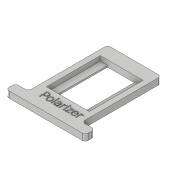
# Autodesk Inventor part: 00_Polarizationfilter_Holder
Saved by Autodesk Inventor 2019.4 (Build 234330000, 330)
## iProperties
Created: 2021-10-22
Part Number: 00_Polarizationfilter_Holder
Material: Generic
Document SubType Name: Modeling
Designer: diederichbenedict
Density: 1 g/cm^3
Appearance: Default
Author: diederichbenedict
Autodesk Inventor part; units mm, degrees
ref_plane "YZ Plane" through (0, 0, 0) normal (1, 0, 0) x (0, 1, 0)
ref_plane "XZ Plane" through (0, 0, 0) normal (0, 1, 0) x (-1, 0, 0)
ref_plane "XY Plane" through (0, 0, 0) normal (0, 0, 1) x (1, 0, 0)
sketch "Sketch1" plane through (0, 0, 0) normal (0, 1, 0) x (-1, 0, 0)
  line L0 (-16.92, 25) -> (16.92, 25)
  line L1 (16.92, 25) -> (16.92, -25)
  line L2 (16.92, -25) -> (-16.92, -25)
  line L3 (-16.92, -25) -> (-16.92, 25)
  line L4 (-16.92, 25) -> (16.92, -25) construction
  line L5 (16.92, 25) -> (-16.92, -25) construction
  line L6 (8.92, -17) -> (8.92, 17)
  line L7 (8.92, 17) -> (-8.92, 17)
  line L8 (-8.92, 17) -> (-8.92, -17)
  line L9 (-8.92, -17) -> (8.92, -17)
  line L10 (-25, 31) -> (25, 31)
  line L11 (25, 31) -> (25, 25)
  line L12 (25, 25) -> (-25, 25)
  line L13 (-25, 25) -> (-25, 31)
  line L14 (-25, 31) -> (25, 25) construction
  line L15 (25, 31) -> (-25, 25) construction
  point P0 (0, 0)
  point P1 (0, 28)
  point P2 (0, 25)
  dimension "d0" = 33.84
  dimension "d1" = 50
  dimension "d2" = 8
  dimension "d3" = 50
  dimension "d4" = 6
  constraints: 32 end point, 6 midpoint, 6 parallel, 3 perpendicular, 2 horizontal, 3 other
  measures "d0" distance of L1.end L2.end
  measures "d1" distance of L0.end L1.end
  measures "d2" distance between parallel lines of L1 L6
  measures "d3" distance of L11.end L12.end
  measures "d4" distance of L10.end L11.end
extrude "Extrusion1" add sketch "Sketch1" along normal blind 4
sketch "Sketch2" plane through (0, 4, 0) normal (0, 1, 0) x (1, 0, 0)
  line L0 (-8.92, 17) -> (8.92, 17) projected
  line L1 (8.92, 17) -> (8.92, -17) projected
  line L2 (8.92, -17) -> (-8.92, -17) projected
  line L3 (-8.92, -17) -> (-8.92, 17) projected
  line L4 (25, -25) -> (16.92, -25) projected
  line L5 (16.92, -25) -> (16.92, 25) projected
  line L6 (16.92, 25) -> (-16.92, 25) projected
  line L7 (-16.92, 25) -> (-16.92, -25) projected
  line L8 (-16.92, -25) -> (-25, -25) projected
  line L9 (-25, -25) -> (-25, -31) projected
  line L10 (-25, -31) -> (25, -31) projected
  line L11 (25, -31) -> (25, -25) projected
  line L12 (13.5, 17) -> (-13.5, 17)
  line L13 (-13.5, 17) -> (-13.5, -17)
  line L14 (-13.5, -17) -> (13.5, -17)
  line L15 (13.5, -17) -> (13.5, 17)
  line L16 (13.5, 17) -> (-13.5, -17) construction
  line L17 (-13.5, 17) -> (13.5, -17) construction
  point P0 (0, 0)
  dimension "d7" = 27
  dimension "d8" = 34
  constraints: 12 end point, 2 midpoint, 2 parallel, 1 horizontal, 1 perpendicular
  measures "d7" distance of L14.end L13.end
  measures "d8" distance of L13.end L12.end
extrude "Extrusion2" cut sketch "Sketch2" against normal blind 3 contours L3 L14 L13 L12 | L12 L15 L14 L1
sketch "Sketch3" plane through (0, 4, 0) normal (0, 1, 0) x (1, 0, 0)
  line L0 (-11.1728, -19.2539) -> (14.053, -19.2539) construction
  line L1 (14.053, -19.2539) -> (14.053, -24.441) construction
  line L2 (14.053, -24.441) -> (-11.1728, -24.441) construction
  line L3 (-11.1728, -24.441) -> (-11.1728, -19.2539) construction
  spline S0 degree 2 poles (-7.603, -20.9382) (-7.603, -21.2538) (-7.8278, -21.8218) (-8.029, -22.019) knots 0 0 0 1 2 2 2
  spline S1 degree 2 poles (-8.029, -22.019) (-8.2814, -22.2675) (-8.9639, -22.5239) (-9.4846, -22.5239) knots 0 0 0 1 2 2 2
  line L4 (-9.4846, -22.5239) -> (-10.0329, -22.5239)
  line L5 (-10.0329, -22.5239) -> (-10.0329, -24.3385)
  line L6 (-10.0329, -24.3385) -> (-10.6798, -24.3385)
  line L7 (-10.6798, -24.3385) -> (-10.6798, -19.4708)
  line L8 (-10.6798, -19.4708) -> (-9.4569, -19.4708)
  spline S2 degree 2 poles (-9.4569, -19.4708) (-9.023, -19.4708) (-8.4156, -19.6128) (-8.1828, -19.7745) knots 0 0 0 1 2 2 2
  spline S3 degree 2 poles (-8.1828, -19.7745) (-7.9107, -19.9599) (-7.603, -20.5319) (-7.603, -20.9382) knots 0 0 0 1 2 2 2
  spline S4 degree 2 poles (-8.2775, -20.9579) (-8.2775, -20.7055) (-8.4511, -20.3347) (-8.6286, -20.2163) knots 0 0 0 1 2 2 2
  spline S5 degree 2 poles (-8.6286, -20.2163) (-8.7824, -20.1138) (-9.1927, -20.0309) (-9.4964, -20.0309) knots 0 0 0 1 2 2 2
  line L9 (-9.4964, -20.0309) -> (-10.0329, -20.0309)
  line L10 (-10.0329, -20.0309) -> (-10.0329, -21.9717)
  line L11 (-10.0329, -21.9717) -> (-9.5911, -21.9717)
  spline S6 degree 2 poles (-9.5911, -21.9717) (-9.1966, -21.9717) (-8.7114, -21.8455) (-8.5536, -21.6798) knots 0 0 0 1 2 2 2
  spline S7 degree 2 poles (-8.5536, -21.6798) (-8.4077, -21.5338) (-8.2775, -21.1907) (-8.2775, -20.9579) knots 0 0 0 1 2 2 2
  spline S8 degree 2 poles (-4.0331, -22.5121) (-4.0331, -23.4351) (-4.9206, -24.441) (-5.6622, -24.441) knots 0 0 0 1 2 2 2
  spline S9 degree 2 poles (-5.6622, -24.441) (-6.4235, -24.441) (-7.2953, -23.4036) (-7.2953, -22.5121) knots 0 0 0 1 2 2 2
  spline S10 degree 2 poles (-7.2953, -22.5121) (-7.2953, -21.597) (-6.3959, -20.5832) (-5.6622, -20.5832) knots 0 0 0 1 2 2 2
  spline S11 degree 2 poles (-5.6622, -20.5832) (-4.9206, -20.5832) (-4.0331, -21.593) (-4.0331, -22.5121) knots 0 0 0 1 2 2 2
  spline S12 degree 2 poles (-4.6682, -22.5121) (-4.6682, -21.8021) (-5.1849, -21.1118) (-5.6622, -21.1118) knots 0 0 0 1 2 2 2
  spline S13 degree 2 poles (-5.6622, -21.1118) (-6.1395, -21.1118) (-6.6602, -21.8021) (-6.6602, -22.5121) knots 0 0 0 1 2 2 2
  spline S14 degree 2 poles (-6.6602, -22.5121) (-6.6602, -23.2024) (-6.1395, -23.9124) (-5.6622, -23.9124) knots 0 0 0 1 2 2 2
  spline S15 degree 2 poles (-5.6622, -23.9124) (-5.1889, -23.9124) (-4.6682, -23.2143) (-4.6682, -22.5121) knots 0 0 0 1 2 2 2
  line L12 (-2.7748, -24.3385) -> (-3.3901, -24.3385)
  line L13 (-3.3901, -24.3385) -> (-3.3901, -19.2539)
  line L14 (-3.3901, -19.2539) -> (-2.7748, -19.2539)
  line L15 (-2.7748, -19.2539) -> (-2.7748, -24.3385)
  spline S16 degree 2 poles (0.164, -23.9519) (0.089, -24.0071) (-0.1634, -24.2043) (-0.2818, -24.2635) knots 0 0 0 1 2 2 2
  spline S17 degree 2 poles (-0.2818, -24.2635) (-0.4435, -24.3503) (-0.7472, -24.441) (-1.0234, -24.441) knots 0 0 0 1 2 2 2
  spline S18 degree 2 poles (-1.0234, -24.441) (-1.2482, -24.441) (-1.6545, -24.2714) (-1.8083, -24.1176) knots 0 0 0 1 2 2 2
  spline S19 degree 2 poles (-1.8083, -24.1176) (-1.9543, -23.9677) (-2.1318, -23.5259) (-2.1318, -23.2813) knots 0 0 0 1 2 2 2
  spline S20 degree 2 poles (-2.1318, -23.2813) (-2.1318, -22.9026) (-1.8123, -22.3662) (-1.4651, -22.2123) knots 0 0 0 1 2 2 2
  spline S21 degree 2 poles (-1.4651, -22.2123) (-1.1575, -22.0703) (-0.3212, -21.9638) (0.164, -21.9362) knots 0 0 0 1 2 2 2
  line L16 (0.164, -21.9362) -> (0.164, -21.8179)
  spline S22 degree 2 poles (0.164, -21.8179) (0.164, -21.6048) (0.0338, -21.3406) (-0.0845, -21.2656) knots 0 0 0 1 2 2 2
  spline S23 degree 2 poles (-0.0845, -21.2656) (-0.2029, -21.1907) (-0.5421, -21.1433) (-0.7236, -21.1433) knots 0 0 0 1 2 2 2
  spline S24 degree 2 poles (-0.7236, -21.1433) (-0.9366, -21.1433) (-1.5125, -21.2696) (-1.8004, -21.3918) knots 0 0 0 1 2 2 2
  line L17 (-1.8004, -21.3918) -> (-1.8359, -21.3918)
  line L18 (-1.8359, -21.3918) -> (-1.8359, -20.7646)
  spline S25 degree 2 poles (-1.8359, -20.7646) (-1.6663, -20.7173) (-1.0312, -20.599) (-0.7196, -20.599) knots 0 0 0 1 2 2 2
  spline S26 degree 2 poles (-0.7196, -20.599) (-0.3409, -20.599) (0.1758, -20.7173) (0.3809, -20.8711) knots 0 0 0 1 2 2 2
  spline S27 degree 2 poles (0.3809, -20.8711) (0.5821, -21.021) (0.7793, -21.4983) (0.7793, -21.8415) knots 0 0 0 1 2 2 2
  line L19 (0.7793, -21.8415) -> (0.7793, -24.3385)
  line L20 (0.7793, -24.3385) -> (0.164, -24.3385)
  line L21 (0.164, -24.3385) -> (0.164, -23.9519)
  line L22 (0.164, -23.4391) -> (0.164, -22.4253)
  spline S28 degree 2 poles (0.164, -22.4253) (-0.0569, -22.4451) (-0.7236, -22.5121) (-0.9326, -22.5752) knots 0 0 0 1 2 2 2
  spline S29 degree 2 poles (-0.9326, -22.5752) (-1.1772, -22.6502) (-1.4967, -22.9618) (-1.4967, -23.2379) knots 0 0 0 1 2 2 2
  spline S30 degree 2 poles (-1.4967, -23.2379) (-1.4967, -23.5535) (-1.1417, -23.873) (-0.8025, -23.873) knots 0 0 0 1 2 2 2
  spline S31 degree 2 poles (-0.8025, -23.873) (-0.5145, -23.873) (-0.0411, -23.6245) (0.164, -23.4391) knots 0 0 0 1 2 2 2
  line L23 (3.58, -21.3445) -> (3.5485, -21.3445)
  spline S32 degree 2 poles (3.5485, -21.3445) (3.4775, -21.3248) (3.3236, -21.3169) (3.2171, -21.3169) knots 0 0 0 1 2 2 2
  spline S33 degree 2 poles (3.2171, -21.3169) (2.9686, -21.3169) (2.4795, -21.5338) (2.2586, -21.7469) knots 0 0 0 1 2 2 2
  line L24 (2.2586, -21.7469) -> (2.2586, -24.3385)
  line L25 (2.2586, -24.3385) -> (1.6432, -24.3385)
  line L26 (1.6432, -24.3385) -> (1.6432, -20.6858)
  line L27 (1.6432, -20.6858) -> (2.2586, -20.6858)
  line L28 (2.2586, -20.6858) -> (2.2586, -21.2301)
  spline S34 degree 2 poles (2.2586, -21.2301) (2.5939, -20.9303) (3.0948, -20.6858) (3.3315, -20.6858) knots 0 0 0 1 2 2 2
  spline S35 degree 2 poles (3.3315, -20.6858) (3.4262, -20.6858) (3.5208, -20.6936) (3.58, -20.7055) knots 0 0 0 1 2 2 2
  line L29 (3.58, -20.7055) -> (3.58, -21.3445)
  line L30 (4.6845, -24.3385) -> (4.0691, -24.3385)
  line L31 (4.0691, -24.3385) -> (4.0691, -20.6858)
  line L32 (4.0691, -20.6858) -> (4.6845, -20.6858)
  line L33 (4.6845, -20.6858) -> (4.6845, -24.3385)
  line L34 (4.7279, -20.0783) -> (4.0297, -20.0783)
  line L35 (4.0297, -20.0783) -> (4.0297, -19.4393)
  line L36 (4.0297, -19.4393) -> (4.7279, -19.4393)
  line L37 (4.7279, -19.4393) -> (4.7279, -20.0783)
  line L38 (7.9862, -24.3385) -> (5.3038, -24.3385)
  line L39 (5.3038, -24.3385) -> (5.3038, -23.8809)
  line L40 (5.3038, -23.8809) -> (7.213, -21.1907)
  line L41 (7.213, -21.1907) -> (5.3827, -21.1907)
  line L42 (5.3827, -21.1907) -> (5.3827, -20.6858)
  line L43 (5.3827, -20.6858) -> (7.9506, -20.6858)
  line L44 (7.9506, -20.6858) -> (7.9506, -21.1236)
  line L45 (7.9506, -21.1236) -> (6.0336, -23.8217)
  line L46 (6.0336, -23.8217) -> (7.9862, -23.8217)
  line L47 (7.9862, -23.8217) -> (7.9862, -24.3385)
  spline S36 degree 2 poles (10.1478, -24.4213) (9.2721, -24.4213) (8.3096, -23.4391) (8.3096, -22.5318) knots 0 0 0 1 2 2 2
  spline S37 degree 2 poles (8.3096, -22.5318) (8.3096, -21.6403) (9.2445, -20.5832) (9.9979, -20.5832) knots 0 0 0 1 2 2 2
  spline S38 degree 2 poles (9.9979, -20.5832) (10.3371, -20.5832) (10.8618, -20.7804) (11.0551, -20.9895) knots 0 0 0 1 2 2 2
  spline S39 degree 2 poles (11.0551, -20.9895) (11.2523, -21.1986) (11.4614, -21.8021) (11.4614, -22.2399) knots 0 0 0 1 2 2 2
  line L48 (11.4614, -22.2399) -> (11.4614, -22.5752)
  line L49 (11.4614, -22.5752) -> (8.9329, -22.5752)
  spline S40 degree 2 poles (8.9329, -22.5752) (8.9329, -23.2103) (9.5719, -23.8848) (10.1399, -23.8848) knots 0 0 0 1 2 2 2
  spline S41 degree 2 poles (10.1399, -23.8848) (10.3411, -23.8848) (10.7316, -23.7941) (10.8894, -23.7231) knots 0 0 0 1 2 2 2
  spline S42 degree 2 poles (10.8894, -23.7231) (11.0551, -23.6442) (11.2839, -23.5062) (11.3588, -23.443) knots 0 0 0 1 2 2 2
  line L50 (11.3588, -23.443) -> (11.3943, -23.443)
  line L51 (11.3943, -23.443) -> (11.3943, -24.1136)
  spline S43 degree 2 poles (11.3943, -24.1136) (11.2878, -24.157) (10.9643, -24.2832) (10.8381, -24.3187) knots 0 0 0 1 2 2 2
  spline S44 degree 2 poles (10.8381, -24.3187) (10.6606, -24.37) (10.3687, -24.4213) (10.1478, -24.4213) knots 0 0 0 1 2 2 2
  spline S45 degree 2 poles (10.8618, -22.1058) (10.8539, -21.8573) (10.7513, -21.4944) (10.6527, -21.3721) knots 0 0 0 1 2 2 2
  spline S46 degree 2 poles (10.6527, -21.3721) (10.5462, -21.2341) (10.2109, -21.0881) (9.9624, -21.0881) knots 0 0 0 1 2 2 2
  spline S47 degree 2 poles (9.9624, -21.0881) (9.7178, -21.0881) (9.3747, -21.2341) (9.2327, -21.3761) knots 0 0 0 1 2 2 2
  spline S48 degree 2 poles (9.2327, -21.3761) (9.0946, -21.522) (8.9526, -21.8731) (8.9329, -22.1058) knots 0 0 0 1 2 2 2
  line L52 (8.9329, -22.1058) -> (10.8618, -22.1058)
  line L53 (14.0214, -21.3445) -> (13.9899, -21.3445)
  spline S49 degree 2 poles (13.9899, -21.3445) (13.9189, -21.3248) (13.765, -21.3169) (13.6585, -21.3169) knots 0 0 0 1 2 2 2
  spline S50 degree 2 poles (13.6585, -21.3169) (13.41, -21.3169) (12.9209, -21.5338) (12.7, -21.7469) knots 0 0 0 1 2 2 2
  line L54 (12.7, -21.7469) -> (12.7, -24.3385)
  line L55 (12.7, -24.3385) -> (12.0846, -24.3385)
  line L56 (12.0846, -24.3385) -> (12.0846, -20.6858)
  line L57 (12.0846, -20.6858) -> (12.7, -20.6858)
  line L58 (12.7, -20.6858) -> (12.7, -21.2301)
  spline S51 degree 2 poles (12.7, -21.2301) (13.0353, -20.9303) (13.5362, -20.6858) (13.7729, -20.6858) knots 0 0 0 1 2 2 2
  spline S52 degree 2 poles (13.7729, -20.6858) (13.8676, -20.6858) (13.9622, -20.6936) (14.0214, -20.7055) knots 0 0 0 1 2 2 2
  line L59 (14.0214, -20.7055) -> (14.0214, -21.3445)
  point P0 (0, 0)
  constraints: 2 other
extrude "Extrusion3" cut sketch "Sketch3" against normal blind 1
fillet "Fillet1" radius 2 8 edges at (25, 2, 31) (25, 2, 25) (-25, 2, 31) (-25, 2, 25) (-16.92, 2, 25) (-16.92, 2, -25) (16.92, 2, -25) (16.92, 2, 25)
body "Solid1"
